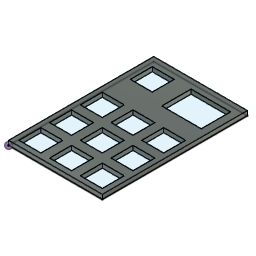
macro pad inside v2 (Autodesk Fusion 360 design; units mm, degrees)
Autodesk Fusion 360 part; units mm, degrees
sketch "Esquisse1" plane through (0, 0, 0) normal (0, 0, 1) x (1, 0, 0)
  line L0 (0, 0) -> (64, 0)
  line L1 (64, 0) -> (64, 99.2)
  line L2 (64, 99.2) -> (0, 99.2)
  line L3 (0, 99.2) -> (0, 0)
  dimension "d1" = 64
  dimension "d2" = 99.2
  constraint horizontal L0
  constraint vertical L1
  constraint horizontal L2
  constraint vertical L3
  constraint coincident L0.start L3.end
  measures "d1" distance of L0.start L0.end
  measures "d2" distance of L0.start L2.end
extrude "Extrusion12" add sketch "Esquisse1" along normal blind 3 makes body 1
extrude "Extrusion1" add sketch "Esquisse1" along normal blind 3 separate body makes body 2
sketch "Esquisse2" plane through (0, 0, 3) normal (0, 0, 1) x (-1, 0, 0)
  line L0 (0, -99.2) -> (0, 0)
  line L1 (0, 0) -> (-64, 0)
  line L2 (-64, 0) -> (-64, -99.2)
  line L3 (-64, -99.2) -> (0, -99.2)
  line L4 (-7.5, -92.7) -> (-22.5, -92.7)
  line L5 (-22.5, -92.7) -> (-22.5, -77.7)
  line L6 (-22.5, -77.7) -> (-7.5, -77.7)
  line L7 (-7.5, -77.7) -> (-7.5, -92.7)
  dimension "d5" = 15
  dimension "d6" = 15
  dimension "d7" = 6.5
  dimension "d8" = 7.5
  constraint horizontal L4
  constraint vertical L5
  constraint horizontal L6
  constraint vertical L7
  measures "d5" distance of L4.start L4.end
  measures "d6" distance of L4.start L6.end
  measures "d7" distance of L3 L4
  measures "d8" distance of L0 L7
extrude "Extrusion2" cut sketch "Esquisse2" against normal blind 3 contours L4 L5 L6 L7 bodies 2
sketch "Esquisse3" plane through (0, 0, 3) normal (0, 0, 1) x (-1, 0, 0)
  line L0 (0, -99.2) -> (0, 0)
  line L1 (0, 0) -> (-64, 0)
  line L2 (-64, 0) -> (-64, -99.2)
  line L3 (-64, -99.2) -> (0, -99.2)
sketch "Esquisse4" plane through (0, 0, 3) normal (0, 0, 1) x (-1, 0, 0)
  line L0 (-3.5, -18.5) -> (-18.5, -18.5)
  line L1 (-18.5, -18.5) -> (-18.5, -3.5)
  line L2 (-18.5, -3.5) -> (-3.5, -3.5)
  line L3 (-3.5, -3.5) -> (-3.5, -18.5)
  line L4 (0, 0) -> (-64, 0)
  line L5 (0, -99.2) -> (0, 0)
  dimension "d11" = 15
  dimension "d12" = 15
  dimension "d13" = 3.5
  dimension "d14" = 3.5
  constraint horizontal L0
  constraint vertical L1
  constraint horizontal L2
  constraint vertical L3
  measures "d11" distance of L0.start L0.end
  measures "d12" distance of L0.start L2.end
  measures "d13" distance of L2 L4
  measures "d14" distance of L3 L5
extrude "Extrusion3" cut sketch "Esquisse4" against normal blind 3 bodies 2
sketch "Esquisse5" plane through (0, 0, 3) normal (0, 0, 1) x (-1, 0, 0)
  line L0 (-24.5, -18.5) -> (-39.5, -18.5)
  line L1 (-39.5, -18.5) -> (-39.5, -3.5)
  line L2 (-39.5, -3.5) -> (-24.5, -3.5)
  line L3 (-24.5, -3.5) -> (-24.5, -18.5)
  line L4 (0, 0) -> (-64, 0)
  line L5 (0, -99.2) -> (0, 0)
  dimension "d17" = 15
  dimension "d18" = 15
  dimension "d19" = 3.5
  dimension "d20" = 24.5
  constraint horizontal L0
  constraint vertical L1
  constraint horizontal L2
  constraint vertical L3
  measures "d17" distance of L1.end L2.end
  measures "d18" distance of L0.start L2.end
  measures "d19" distance of L2 L4
  measures "d20" distance of L3 L5
extrude "Extrusion4" cut sketch "Esquisse5" against normal blind 3 bodies 2
sketch "Esquisse6" plane through (0, 0, 3) normal (0, 0, 1) x (-1, 0, 0)
  line L0 (-45.5, -18.5) -> (-60.5, -18.5)
  line L1 (-60.5, -18.5) -> (-60.5, -3.5)
  line L2 (-60.5, -3.5) -> (-45.5, -3.5)
  line L3 (-45.5, -3.5) -> (-45.5, -18.5)
  line L4 (0, 0) -> (-64, 0)
  line L5 (-64, 0) -> (-64, -99.2)
  dimension "d23" = 15
  dimension "d24" = 15
  dimension "d25" = 3.5
  dimension "d26" = 3.5
  constraint horizontal L0
  constraint vertical L1
  constraint horizontal L2
  constraint vertical L3
  measures "d23" distance of L0.start L0.end
  measures "d24" distance of L0.end L1.end
  measures "d25" distance of L2 L4
  measures "d26" distance of L1 L5
extrude "Extrusion5" cut sketch "Esquisse6" against normal blind 3 bodies 2
sketch "Esquisse7" plane through (0, 0, 3) normal (0, 0, 1) x (-1, 0, 0)
  line L0 (-3.5, -39.5) -> (-18.5, -39.5)
  line L1 (-18.5, -39.5) -> (-18.5, -24.5)
  line L2 (-18.5, -24.5) -> (-3.5, -24.5)
  line L3 (-3.5, -24.5) -> (-3.5, -39.5)
  line L4 (0, 0) -> (-64, 0)
  line L5 (0, -99.2) -> (0, 0)
  dimension "d29" = 15
  dimension "d30" = 15
  dimension "d31" = 24.5
  dimension "d32" = 3.5
  constraint horizontal L0
  constraint vertical L1
  constraint horizontal L2
  constraint vertical L3
  measures "d29" distance of L1.end L2.end
  measures "d30" distance of L0.start L2.end
  measures "d31" distance of L2 L4
  measures "d32" distance of L3 L5
extrude "Extrusion6" cut sketch "Esquisse7" against normal blind 3 bodies 2
sketch "Esquisse8" plane through (0, 0, 3) normal (0, 0, 1) x (-1, 0, 0)
  line L0 (-24.5, -39.5) -> (-39.5, -39.5)
  line L1 (-39.5, -39.5) -> (-39.5, -24.5)
  line L2 (-39.5, -24.5) -> (-24.5, -24.5)
  line L3 (-24.5, -24.5) -> (-24.5, -39.5)
  line L4 (0, -99.2) -> (0, 0)
  line L5 (0, 0) -> (-64, 0)
  line L6 (-45.5, -39.5) -> (-60.5, -39.5)
  line L7 (-60.5, -39.5) -> (-60.5, -24.5)
  line L8 (-60.5, -24.5) -> (-45.5, -24.5)
  line L9 (-45.5, -24.5) -> (-45.5, -39.5)
  line L10 (-64, 0) -> (-64, -99.2)
  dimension "d35" = 15
  dimension "d36" = 15
  dimension "d37" = 24.5
  dimension "d38" = 24.5
  dimension "d39" = 15
  dimension "d40" = 15
  dimension "d41" = 24.5
  dimension "d42" = 3.5
  constraint horizontal L0
  constraint vertical L1
  constraint horizontal L2
  constraint vertical L3
  constraint horizontal L6
  constraint vertical L7
  constraint horizontal L8
  constraint vertical L9
  measures "d35" distance of L0.start L2.end
  measures "d36" distance of L1.end L2.end
  measures "d37" distance of L3 L4
  measures "d38" distance of L2 L5
  measures "d39" distance of L7.end L8.end
  measures "d40" distance of L6.start L8.end
  measures "d41" distance of L5 L8
  measures "d42" distance of L7 L10
extrude "Extrusion7" cut sketch "Esquisse8" against normal blind 3 bodies 2
sketch "Esquisse9" plane through (0, 0, 3) normal (0, 0, 1) x (-1, 0, 0)
  line L0 (-3.5, -60.5) -> (-18.5, -60.5)
  line L1 (-18.5, -60.5) -> (-18.5, -45.5)
  line L2 (-18.5, -45.5) -> (-3.5, -45.5)
  line L3 (-3.5, -45.5) -> (-3.5, -60.5)
  line L4 (0, -99.2) -> (0, 0)
  line L5 (0, 0) -> (-64, 0)
  dimension "d45" = 15
  dimension "d46" = 15
  dimension "d47" = 3.5
  dimension "d48" = 45.5
  constraint horizontal L0
  constraint vertical L1
  constraint horizontal L2
  constraint vertical L3
  measures "d45" distance of L0.start L2.end
  measures "d46" distance of L1.end L2.end
  measures "d47" distance of L3 L4
  measures "d48" distance of L2 L5
extrude "Extrusion8" cut sketch "Esquisse9" against normal blind 3 bodies 2
sketch "Esquisse10" plane through (0, 0, 3) normal (0, 0, 1) x (-1, 0, 0)
  line L0 (-24.5, -60.5) -> (-39.5, -60.5)
  line L1 (-39.5, -60.5) -> (-39.5, -45.5)
  line L2 (-39.5, -45.5) -> (-24.5, -45.5)
  line L3 (-24.5, -45.5) -> (-24.5, -60.5)
  line L4 (0, -99.2) -> (0, 0)
  line L5 (0, 0) -> (-64, 0)
  dimension "d51" = 15
  dimension "d52" = 15
  dimension "d53" = 24.5
  dimension "d54" = 45.5
  constraint horizontal L0
  constraint vertical L1
  constraint horizontal L2
  constraint vertical L3
  measures "d51" distance of L0.start L0.end
  measures "d52" distance of L0.start L2.end
  measures "d53" distance of L3 L4
  measures "d54" distance of L2 L5
extrude "Extrusion9" cut sketch "Esquisse10" against normal blind 3 bodies 2
sketch "Esquisse11" plane through (0, 0, 3) normal (0, 0, 1) x (-1, 0, 0)
  line L0 (-45.5, -60.5) -> (-60.5, -60.5)
  line L1 (-60.5, -60.5) -> (-60.5, -45.5)
  line L2 (-60.5, -45.5) -> (-45.5, -45.5)
  line L3 (-45.5, -45.5) -> (-45.5, -60.5)
  line L4 (0, 0) -> (-64, 0)
  line L5 (-64, 0) -> (-64, -99.2)
  dimension "d57" = 15
  dimension "d58" = 15
  dimension "d59" = 45.5
  dimension "d60" = 3.5
  constraint horizontal L0
  constraint vertical L1
  constraint horizontal L2
  constraint vertical L3
  measures "d57" distance of L0.start L0.end
  measures "d58" distance of L0.end L1.end
  measures "d59" distance of L2 L4
  measures "d60" distance of L1 L5
extrude "Extrusion10" cut sketch "Esquisse11" against normal blind 3 bodies 2
delete_face "DeleteFace1" 4 faces at (12.5, 92.7, 2) (7.5, 82.7, 2) (22.5, 87.7, 2) (17.5, 77.7, 2) on bodies 2
sketch "Esquisse15" plane through (0, 0, 3) normal (0, 0, 1) x (-1, 0, 0)
  line L0 (-60.5, -3.5) -> (-45.5, -3.5)
  line L1 (-45.5, -3.5) -> (-45.5, -18.5)
  line L2 (-45.5, -18.5) -> (-60.5, -18.5)
  line L3 (-60.5, -18.5) -> (-60.5, -3.5)
  line L4 (-39.5, -18.5) -> (-24.5, -18.5)
  line L5 (-24.5, -18.5) -> (-24.5, -3.5)
  line L6 (-24.5, -3.5) -> (-39.5, -3.5)
  line L7 (-39.5, -3.5) -> (-39.5, -18.5)
  line L8 (-60.5, -39.5) -> (-45.5, -39.5)
  line L9 (-45.5, -39.5) -> (-45.5, -24.5)
  line L10 (-45.5, -24.5) -> (-60.5, -24.5)
  line L11 (-60.5, -24.5) -> (-60.5, -39.5)
  line L12 (-39.5, -24.5) -> (-24.5, -24.5)
  line L13 (-24.5, -24.5) -> (-24.5, -39.5)
  line L14 (-24.5, -39.5) -> (-39.5, -39.5)
  line L15 (-39.5, -39.5) -> (-39.5, -24.5)
  line L16 (-18.5, -3.5) -> (-3.5, -3.5)
  line L17 (-3.5, -3.5) -> (-3.5, -18.5)
  line L18 (-3.5, -18.5) -> (-18.5, -18.5)
  line L19 (-18.5, -18.5) -> (-18.5, -3.5)
  line L20 (-60.5, -45.5) -> (-45.5, -45.5)
  line L21 (-45.5, -45.5) -> (-45.5, -60.5)
  line L22 (-45.5, -60.5) -> (-60.5, -60.5)
  line L23 (-60.5, -60.5) -> (-60.5, -45.5)
  line L24 (-39.5, -60.5) -> (-24.5, -60.5)
  line L25 (-24.5, -60.5) -> (-24.5, -45.5)
  line L26 (-24.5, -45.5) -> (-39.5, -45.5)
  line L27 (-39.5, -45.5) -> (-39.5, -60.5)
  line L28 (-18.5, -60.5) -> (-3.5, -60.5)
  line L29 (-3.5, -60.5) -> (-3.5, -45.5)
  line L30 (-3.5, -45.5) -> (-18.5, -45.5)
  line L31 (-18.5, -45.5) -> (-18.5, -60.5)
  line L32 (-18.5, -39.5) -> (-3.5, -39.5)
  line L33 (-3.5, -39.5) -> (-3.5, -24.5)
  line L34 (-3.5, -24.5) -> (-18.5, -24.5)
  line L35 (-18.5, -24.5) -> (-18.5, -39.5)
  point P0 (-45.5, -18.5)
  point P1 (-60.5, -18.5)
  point P2 (-60.5, -3.5)
  point P3 (-39.5, -18.5)
  point P4 (-24.5, -18.5)
  point P5 (-24.5, -3.5)
  point P6 (-60.5, -39.5)
  point P7 (-45.5, -39.5)
  point P8 (-45.5, -24.5)
  point P9 (-39.5, -24.5)
  point P10 (-24.5, -24.5)
  point P11 (-24.5, -39.5)
  point P12 (-18.5, -3.5)
  point P13 (-3.5, -3.5)
  point P14 (-3.5, -18.5)
  point P15 (-60.5, -45.5)
  point P16 (-45.5, -45.5)
  point P17 (-45.5, -60.5)
  point P18 (-39.5, -60.5)
  point P19 (-24.5, -60.5)
  point P20 (-24.5, -45.5)
  point P21 (-18.5, -60.5)
  point P22 (-3.5, -45.5)
  point P23 (-18.5, -39.5)
  point P24 (-3.5, -24.5)
  constraint horizontal L0
  constraint vertical L1
  constraint horizontal L2
  constraint vertical L3
  constraint coincident P0 L1.end
  constraint coincident P1 L2.end
  constraint coincident P2 L0.start
  constraint horizontal L4
  constraint vertical L5
  constraint horizontal L6
  constraint vertical L7
  constraint coincident P3 L4.start
  constraint coincident P4 L4.end
  constraint coincident P5 L5.end
  constraint horizontal L8
  constraint vertical L9
  constraint horizontal L10
  constraint vertical L11
  constraint coincident P6 L8.start
  constraint coincident P7 L8.end
  constraint coincident P8 L9.end
  constraint horizontal L12
  constraint vertical L13
  constraint horizontal L14
  constraint vertical L15
  constraint coincident P9 L12.start
  constraint coincident P10 L12.end
  constraint coincident P11 L13.end
  constraint horizontal L16
  constraint vertical L17
  constraint horizontal L18
  constraint vertical L19
  constraint coincident P12 L16.start
  constraint coincident P13 L16.end
  constraint coincident P14 L17.end
  constraint horizontal L20
  constraint vertical L21
  constraint horizontal L22
  constraint vertical L23
  constraint coincident P15 L20.start
  constraint coincident P16 L20.end
  constraint coincident P17 L21.end
  constraint horizontal L24
  constraint vertical L25
  constraint horizontal L26
  constraint vertical L27
  constraint coincident P18 L24.start
  constraint coincident P19 L24.end
  constraint coincident P20 L25.end
  constraint horizontal L28
  constraint vertical L29
  constraint horizontal L30
  constraint vertical L31
  constraint coincident P21 L28.start
  constraint coincident P22 L29.end
  constraint horizontal L32
  constraint vertical L33
  constraint horizontal L34
  constraint vertical L35
  constraint coincident P23 L32.start
  constraint coincident P24 L33.end
extrude "Extrusion14" cut sketch "Esquisse15" against normal blind 3 bodies 1
sketch "Esquisse16" plane through (0, 0, 3) normal (0, 0, 1) x (-1, 0, 0)
  line L0 (-5.5, -92.7) -> (-20.5, -92.7)
  line L1 (-20.5, -92.7) -> (-20.5, -77.7)
  line L2 (-20.5, -77.7) -> (-5.5, -77.7)
  line L3 (-5.5, -77.7) -> (-5.5, -92.7)
  line L4 (-64, -99.2) -> (0, -99.2)
  line L5 (0, -99.2) -> (0, 0)
  line L6 (-32, -92.7) -> (-59, -92.7)
  line L7 (-59, -92.7) -> (-59, -72.7)
  line L8 (-59, -72.7) -> (-32, -72.7)
  line L9 (-32, -72.7) -> (-32, -92.7)
  line L10 (-64, 0) -> (-64, -99.2)
  dimension "d80" = 15
  dimension "d81" = 15
  dimension "d82" = 6.5
  dimension "d83" = 5.5
  dimension "d84" = 20
  dimension "d85" = 6.5
  dimension "d86" = 27
  dimension "d87" = 5
  constraint horizontal L0
  constraint vertical L1
  constraint horizontal L2
  constraint vertical L3
  constraint horizontal L6
  constraint vertical L7
  constraint horizontal L8
  constraint vertical L9
  measures "d80" distance of L0.start L0.end
  measures "d81" distance of L0.end L1.end
  measures "d82" distance of L0 L4
  measures "d83" distance of L3 L5
  measures "d84" distance of L6.end L7.end
  measures "d85" distance of L4 L6
  measures "d86" distance of L6.start L6.end
  measures "d87" distance of L7 L10
extrude "Extrusion15" cut sketch "Esquisse16" against normal blind 3 bodies 1 2
sketch "Esquisse12" plane through (0, 0, 3) normal (0, 0, 1) x (-1, 0, 0)
  line L0 (-29.5, -96.2) -> (-56.5, -96.2)
  line L1 (-56.5, -96.2) -> (-56.5, -74.2)
  line L2 (-56.5, -74.2) -> (-29.5, -74.2)
  line L3 (-29.5, -74.2) -> (-29.5, -96.2)
  line L4 (-64, 0) -> (-64, -99.2)
  line L5 (-64, -99.2) -> (0, -99.2)
  dimension "d63" = 7.5
  dimension "d64" = 22
  dimension "d65" = 27
  dimension "d66" = 3
  constraint horizontal L0
  constraint vertical L1
  constraint horizontal L2
  constraint vertical L3
  measures "d63" distance of L1 L4
  measures "d64" distance of L0.start L2.end
  measures "d65" distance of L0.start L0.end
  measures "d66" distance of L0 L5
extrude "Extrusion11" [rolled back] along distance -3 taper angle 0
sketch "Esquisse13" plane through (0, 0, 3) normal (0, 0, 1) x (-1, 0, 0)
  line L0 (-64, -99.2) -> (0, -99.2)
  line L1 (0, -99.2) -> (0, 0)
sketch "Esquisse14" plane through (0, 0, 0) normal (0, 0, -1) x (1, 0, 0)
  line L0 (56.5, -74.2) -> (56.5, -96.2)
  line L1 (56.5, -96.2) -> (29.5, -96.2)
  line L2 (29.5, -96.2) -> (29.5, -74.2)
  line L3 (29.5, -74.2) -> (56.5, -74.2)
  line L4 (60.5, -45.5) -> (60.5, -60.5)
  line L5 (60.5, -60.5) -> (45.5, -60.5)
  line L6 (45.5, -60.5) -> (45.5, -45.5)
  line L7 (45.5, -45.5) -> (60.5, -45.5)
  line L8 (39.5, -45.5) -> (39.5, -60.5)
  line L9 (39.5, -60.5) -> (24.5, -60.5)
  line L10 (24.5, -60.5) -> (24.5, -45.5)
  line L11 (24.5, -45.5) -> (39.5, -45.5)
  line L12 (18.5, -45.5) -> (18.5, -60.5)
  line L13 (18.5, -60.5) -> (3.5, -60.5)
  line L14 (3.5, -60.5) -> (3.5, -45.5)
  line L15 (3.5, -45.5) -> (18.5, -45.5)
  line L16 (39.5, -24.5) -> (39.5, -39.5)
  line L17 (39.5, -39.5) -> (24.5, -39.5)
  line L18 (24.5, -39.5) -> (24.5, -24.5)
  line L19 (24.5, -24.5) -> (39.5, -24.5)
  line L20 (60.5, -24.5) -> (60.5, -39.5)
  line L21 (60.5, -39.5) -> (45.5, -39.5)
  line L22 (45.5, -39.5) -> (45.5, -24.5)
  line L23 (45.5, -24.5) -> (60.5, -24.5)
  line L24 (18.5, -24.5) -> (18.5, -39.5)
  line L25 (18.5, -39.5) -> (3.5, -39.5)
  line L26 (3.5, -39.5) -> (3.5, -24.5)
  line L27 (3.5, -24.5) -> (18.5, -24.5)
  line L28 (60.5, -3.5) -> (60.5, -18.5)
  line L29 (60.5, -18.5) -> (45.5, -18.5)
  line L30 (45.5, -18.5) -> (45.5, -3.5)
  line L31 (45.5, -3.5) -> (60.5, -3.5)
  line L32 (39.5, -3.5) -> (39.5, -18.5)
  line L33 (39.5, -18.5) -> (24.5, -18.5)
  line L34 (24.5, -18.5) -> (24.5, -3.5)
  line L35 (24.5, -3.5) -> (39.5, -3.5)
  line L36 (18.5, -3.5) -> (18.5, -18.5)
  line L37 (18.5, -18.5) -> (3.5, -18.5)
  line L38 (3.5, -18.5) -> (3.5, -3.5)
  line L39 (3.5, -3.5) -> (18.5, -3.5)
  line L40 (22.5, -77.7) -> (22.5, -92.7)
  line L41 (22.5, -92.7) -> (7.5, -92.7)
  line L42 (7.5, -92.7) -> (7.5, -77.7)
  line L43 (7.5, -77.7) -> (22.5, -77.7)
  line L44 (0, 0) -> (0, -99.2)
  line L45 (0, -99.2) -> (64, -99.2)
  line L46 (64, -99.2) -> (64, 0)
  line L47 (64, 0) -> (0, 0)
extrude "Extrusion13" [rolled back] along distance -3 taper angle 0
